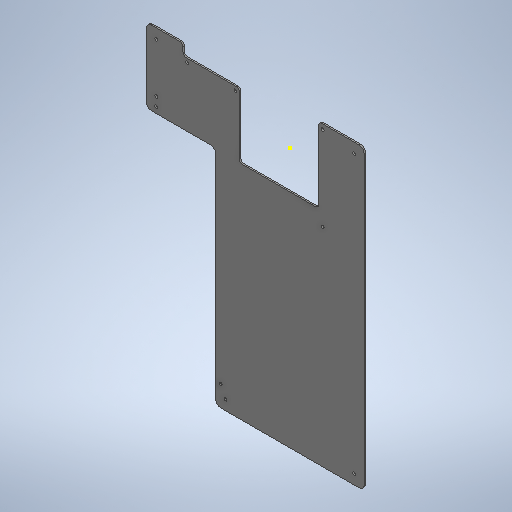
# Autodesk Inventor part: 天板
Saved by Autodesk Inventor 2026.2 (Build 302298010, 298A)
## iProperties
Created: 2026-05-07
Part Number: 天板
Material: 一般
Document SubType Name: Modeling
Designer: Yagis
Density: 1 g/cm^3
Appearance: 既定
Author: Yagis
Autodesk Inventor part; units mm, degrees
ref_plane "YZ Plane" through (0, 0, 0) normal (1, 0, 0) x (0, 1, 0)
ref_plane "XZ Plane" through (0, 0, 0) normal (0, 1, 0) x (-1, 0, 0)
ref_plane "XY Plane" through (0, 0, 0) normal (0, 0, 1) x (1, 0, 0)
sketch "スケッチ2" plane through (0, 0, 0) normal (0, 0, 1) x (1, 0, 0)
  line L0 (-70, 37.5) -> (70, 37.5)
  line L1 (75, 32.5) -> (75, -257.5)
  line L2 (70, -262.5) -> (-70, -262.5)
  line L3 (-75, -183.2657) -> (-75, -42.5)
  arc A0 (75, 32.5) -> (70, 37.5) centre (70, 32.5) ccw
  arc A1 (70, -262.5) -> (75, -257.5) centre (70, -257.5) ccw
  line L4 (-75, -257.5) -> (-75, -183.1423)
  arc A2 (-75, -257.5) -> (-70, -262.5) centre (-70, -257.5) ccw
  line L5 (-70, 37.5) -> (-140, 37.5)
  line L6 (-145, 32.5) -> (-145, -32.5)
  line L7 (-140, -37.5) -> (-80, -37.5)
  arc A3 (-140, 37.5) -> (-145, 32.5) centre (-140, 32.5) ccw
  arc A4 (-145, -32.5) -> (-140, -37.5) centre (-140, -32.5) ccw
  arc A5 (-75, -42.5) -> (-80, -37.5) centre (-80, -42.5) ccw
  point P0 (0, 0)
  point P1 (-75, 37.5)
  point P2 (75, -262.5)
  point P3 (75, 37.5)
  point P4 (-75, -262.5)
  point P5 (-75, 0)
  point P6 (0, 37.5)
  point P7 (0, 0)
  point P8 (-145, 0)
  dimension "d1" = 300
  dimension "d24" = 5
  dimension "d49" = 220
  dimension "d50" = 5
  dimension "d51" = 75
  constraints: 16 end point, 12 point on circle, 12 tangent, 8 point on line, 6 centre point, 3 perpendicular, 2 equal radius, 2 horizontal, 2 midpoint, 1 coincident, 1 collinear, 1 horizontal alignment, 1 parallel, 1 vertical, 1 vertical alignment
  measures "d1" distance of point (75, 37.5) point (75, -262.5)
  measures "d24" radius of A2
  measures "d49" distance from line of L1 point (-145, 0)
  measures "d50" radius of A3
  measures "d51" distance between parallel lines of L7 L5
extrude "押し出し1" add sketch "スケッチ2" along normal blind 1.5
sketch "スケッチ5" plane through (0, 0, 1.5) normal (0, 0, 1) x (1, 0, 0)
  line L0 (70, 37.5) -> (-140, 37.5) projected
  line L1 (75, -257.5) -> (75, 32.5) projected
  line L2 (-70, -262.5) -> (70, -262.5) projected
  line L3 (-145, 32.5) -> (-145, -32.5) projected
  line L4 (-140, -37.5) -> (-80, -37.5) projected
  line L5 (-75, -42.5) -> (-75, -257.5) projected
  point P0 (-135, 27.5)
  point P1 (65, 27.5)
  point P2 (65, -252.5)
  point P3 (-70, 37.5)
  point P4 (-135, -31.5)
  point P5 (-70, -241.5)
  point P6 (33, -52.5)
  point P7 (33, 32.5)
  point P8 (-55, 22.5)
  point P9 (-135, -22.5)
  point P10 (-65, -252.5)
  point P11 (-104, 22.5)
  dimension "d25" = 10
  dimension "d27" = 10
  dimension "d44" = 80
  dimension "d46" = 85
  dimension "d52" = 10
  dimension "d55" = 10
  dimension "d56" = 10
  dimension "d58" = 21
  dimension "d59" = 5
  dimension "d60" = 15
  dimension "d61" = 69
  dimension "d62" = 5
  dimension "d66" = 54
  dimension "d67" = 49
  constraints: 3 vertical alignment, 2 horizontal alignment
  measures "d25" distance from line of point (-135, 27.5) L0
  measures "d27" distance from line of L1 point (65, 27.5)
  measures "d44" horizontal distance of point (-55, 22.5) point (-135, -31.5)
  measures "d46" distance of point (33, -52.5) point (33, 32.5)
  measures "d52" distance from line of L3 point (-135, 27.5)
  measures "d55" distance from line of L2 point (-65, -252.5)
  measures "d56" distance from line of L5 point (-65, -252.5)
  measures "d58" distance from line of L2 point (-70, -241.5)
  measures "d59" distance from line of L5 point (-70, -241.5)
  measures "d60" distance from line of L4 point (-135, -22.5)
  measures "d61" distance from line of L0 point (-135, -31.5)
  measures "d62" distance from line of L0 point (33, 32.5)
  measures "d66" vertical distance of point (-55, 22.5) point (-135, -31.5)
  measures "d67" distance of point (-104, 22.5) point (-55, 22.5)
hole "穴3" at (-135, 27.5, 1.5) at (65, 27.5, 1.5) at (65, -252.5, 1.5) at (-135, -31.5, 1.5) at (-70, -241.5, 1.5) at (-55, 22.5, 1.5) at (33, 32.5, 1.5) at (33, -52.5, 1.5) at (-135, -22.5, 1.5) at (-65, -252.5, 1.5) at (-104, 22.5, 1.5) direction (0, 0, -1) diameter 3 depth 8.1 tip angle 118
sketch "スケッチ6" plane through (0, 0, 1.5) normal (0, 0, 1) x (1, 0, 0)
  point P0 (0, 0)
sketch "スケッチ7" plane through (0, 0, 1.5) normal (0, 0, 1) x (1, 0, 0)
  line L0 (-51, 26.5) -> (-108, 26.5)
  line L1 (-108, 26.5) -> (-108, 37.5)
  line L2 (-108, 37.5) -> (29, 37.5)
  line L3 (29, 37.5) -> (29, -38.5)
  line L4 (-51, 0) -> (-51, 26.5)
  circle A0 centre (-55, 22.5) radius 1.5 projected
  circle A1 centre (-104, 22.5) radius 1.5 projected
  line L5 (70, 37.5) -> (-140, 37.5) projected
  line L6 (29, -38.5) -> (-51, -38.5)
  line L7 (-51, -38.5) -> (-51, 0)
  point P0 (-25.5, 0)
  dimension "d68" = 4
  dimension "d69" = 4
  dimension "d70" = 4
  dimension "d74" = 76
  dimension "d75" = 80
  constraints: 14 end point, 4 perpendicular, 2 horizontal, 1 collinear
  measures "d68" distance from line of L0 A0.centre
  measures "d69" distance from line of L4 A0.centre
  measures "d70" horizontal distance of L0.end A1.centre
  measures "d74" distance of L2.end L3.end
  measures "d75" distance between parallel lines of L3 L7
extrude "押し出し2" cut sketch "スケッチ7" against normal blind 10 contours L0 L1 L2 L3 L6 L7 L4
fillet "フィレット1" radius 3 6 edges at (-108, 26.5, 0.75) (-51, 26.5, 0.75) (-108, 37.5, 0.75) (-51, -38.5, 0.75) (29, -38.5, 0.75) (29, 37.5, 0.75)
